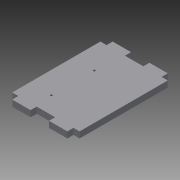
# Autodesk Inventor part: drive-fix
Saved by Autodesk Inventor 2014 (Build 180170000, 170)
## iProperties
Created: 2014-03-02
Part Number: drive-fix
Material: 常规
Document SubType Name: Modeling
Designer: Keshuai
Density: 1 g/cm^3
Appearance: 默认
Author: Keshuai
Autodesk Inventor part; units mm, degrees
ref_plane "YZ Plane" through (0, 0, 0) normal (1, 0, 0) x (0, 1, 0)
ref_plane "XZ Plane" through (0, 0, 0) normal (0, 1, 0) x (-1, 0, 0)
ref_plane "XY Plane" through (0, 0, 0) normal (0, 0, 1) x (1, 0, 0)
sketch "草图1" plane through (0, 0, 0) normal (0, 0, 1) x (1, 0, 0)
  line L0 (-30, 0) -> (-45, 0) projected
  line L1 (-30, 0) -> (-30, 5) projected
  line L2 (-45, 5) -> (-30, 5) projected
  line L3 (-45, 0) -> (-45, 5) projected
  line L4 (0, 0) -> (-15, 0) projected
  line L5 (0, 0) -> (0, 5) projected
  line L6 (-15, 5) -> (0, 5) projected
  line L7 (-15, 0) -> (-15, 5) projected
  line L8 (-42, -72) -> (-37, -72) projected
  line L9 (5, 0) -> (5, -12.0239) projected
  line L10 (5, 0) -> (-50, 0)
  line L11 (-50, 0) -> (-50, -72)
  line L12 (-50, -72) -> (5, -72)
  line L13 (5, -72) -> (5, 0)
  line L14 (-45, -72) -> (-30, -72)
  line L15 (-30, -72) -> (-30, -77)
  line L16 (-30, -77) -> (-45, -77)
  line L17 (-45, -77) -> (-45, -72)
  line L18 (-15, -72) -> (0, -72)
  line L19 (0, -72) -> (0, -77)
  line L20 (0, -77) -> (-15, -77)
  line L21 (-15, -77) -> (-15, -72)
  circle A0 centre (-32, -58) radius 0.85
  circle A1 centre (-32, -23) radius 0.85
  dimension "d0" = 55
  dimension "d1" = 5
  dimension "d2" = 1.7
  dimension "d3" = 14
  dimension "d4" = 37
  dimension "d5" = 1.7
  dimension "d6" = 35
  dimension "d7" = 18
  constraints: 24 end point, 6 parallel, 3 horizontal, 3 perpendicular, 2 centre point, 2 point on line
  measures "d0" distance of L12.end L11.end
  measures "d1" distance of L14.end L15.end
  measures "d2" diameter of A0
  measures "d3" distance from line of L12 A0.centre
  measures "d4" distance from line of L13 A0.centre
  measures "d5" diameter of A1
  measures "d6" distance of A1.centre A0.centre
  measures "d7" distance from line of L11 A0.centre
extrude "拉伸1" add sketch "草图1" along normal blind 5
